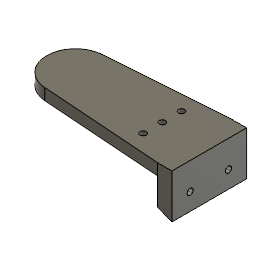
Femur 2 (Autodesk Fusion 360 design; units mm, degrees)
Autodesk Fusion 360 part; units mm, degrees
note: some values were not read from the file. Set by a fixed rule: which sketch regions a step uses.
sketch "Sketch1" plane through (0, 0, 0) normal (0, 1, 0) x (1, 0, 0)
  line L0 (-3.75, 19.5) -> (3.75, 19.5)
  line L1 (3.75, 19.5) -> (3.75, -19.5)
  line L2 (3.75, -19.5) -> (-3.75, -19.5)
  line L3 (-3.75, -19.5) -> (-3.75, 19.5)
  line L4 (-3.75, 19.5) -> (3.75, -19.5) construction
  line L5 (3.75, 19.5) -> (-3.75, -19.5) construction
  circle A0 centre (-66.05, 0) radius 15
  line L6 (-3.75, -19.5) -> (-67.1215, -14.9617)
  line L7 (-3.75, 19.5) -> (-67.1215, 14.9617)
  dimension "d1" = 7.5
  dimension "d2" = 39
  dimension "d4" = 30
  constraint horizontal L0
  constraint perpendicular L0 L1
  constraint parallel L0 L2
  constraint parallel L1 L3
  constraint coincident L4 origin
  constraint coincident L5 origin
  constraint tangent A0 L6
  constraint tangent A0 L7
  constraint coincident A0 L7.end
  constraint coincident A0 L6.end
  measures "d1" distance of L1.end L2.end
  measures "d2" distance of L0.end L1.end
  measures "d4" diameter of A0
extrude "Extrude1" add sketch "Sketch1" along normal blind 6
sketch "Sketch2" plane through (0, 6, 0) normal (0, 1, 0) x (-1, 0, 0)
  line L0 (-3.75, -19.5) -> (3.75, -19.5)
  line L1 (3.75, -19.5) -> (67.1215, -14.9617)
  arc A0 (67.1215, -14.9617) -> (67.1215, 14.9617) centre (66.05, 0) ccw
  line L2 (67.1215, 14.9617) -> (3.75, 19.5)
  line L3 (3.75, 19.5) -> (-3.75, 19.5)
  line L4 (-3.75, 19.5) -> (-3.75, -19.5)
  line L5 (-3.75, 19.5) -> (3.75, 19.5)
  line L6 (3.75, 19.5) -> (3.75, -19.5)
  line L7 (3.75, -19.5) -> (-3.75, -19.5)
  line L8 (-3.75, -19.5) -> (-3.75, 19.5)
  line L9 (-3.75, 19.5) -> (3.75, -19.5) construction
  line L10 (3.75, 19.5) -> (-3.75, -19.5) construction
  dimension "d7" = 7.5
  dimension "d8" = 39
  constraint horizontal L5
  constraint perpendicular L5 L6
  constraint parallel L5 L7
  constraint parallel L6 L8
  constraint coincident L9 origin
  constraint coincident L10 origin
  measures "d7" distance of L0.end L0.start
  measures "d8" distance of L2.end L0.end
extrude "Extrude2" add sketch "Sketch2" against normal blind 20.2 contours L0 L3 L4 L5 L6 L7 L8
sketch "Sketch3" plane through (0, 6, 0) normal (0, 1, 0) x (-1, 0, 0)
  line L0 (3.75, -19.5) -> (67.1215, -14.9617)
  arc A0 (67.1215, -14.9617) -> (67.1215, 14.9617) centre (66.05, 0) ccw
  line L1 (67.1215, 14.9617) -> (3.75, 19.5)
  line L2 (3.75, 19.5) -> (-3.75, 19.5)
  line L3 (-3.75, 19.5) -> (-3.75, -19.5)
  line L4 (-3.75, -19.5) -> (3.75, -19.5)
  circle A1 centre (66.05, 0) radius 4
  dimension "d11" = 8
  constraint concentric A0 A1
  measures "d11" diameter of A1
extrude "Extrude3" add sketch "Sketch3" against normal blind 9 contours A1
sketch "Sketch4" plane through (0, -3, 0) normal (0, -1, 0) x (1, 0, 0)
  circle A0 centre (-66.05, 0) radius 4
  circle A1 centre (-66.05, 0) radius 3
  dimension "d14" = 6
  constraint concentric A0 A1
  measures "d14" diameter of A1
extrude "Extrude4" add sketch "Sketch4" along normal blind 6 contours A1
sketch "Sketch5" plane through (0, 6, 0) normal (0, 1, 0) x (-1, 0, 0)
  line L0 (3.75, -19.5) -> (67.1215, -14.9617)
  arc A0 (67.1215, -14.9617) -> (67.1215, 14.9617) centre (66.05, 0) ccw
  line L1 (67.1215, 14.9617) -> (3.75, 19.5)
  line L2 (3.75, 19.5) -> (-3.75, 19.5)
  line L3 (-3.75, 19.5) -> (-3.75, -19.5)
  line L4 (-3.75, -19.5) -> (3.75, -19.5)
  line L5 (3.75, -19.5) -> (23.6989, -18.0714)
  line L6 (3.75, 19.5) -> (23.6989, 18.0714)
  line L7 (23.6989, 18.0714) -> (23.6989, -18.0714)
  line L8 (23.6989, -18.0714) -> (17.7142, -18.5)
  line L9 (23.6989, 18.0714) -> (17.7142, 18.5)
  line L10 (17.7142, 18.5) -> (17.7142, -18.5)
  line L11 (17.7142, -18.5) -> (23.6989, 18.0714)
  line L12 (23.6989, -18.0714) -> (17.7142, 18.5)
  line L13 (17.7142, 0) -> (23.6989, 0)
  circle A1 centre (20.7416, 0) radius 1.6
  line L14 (20.7416, 0) -> (20.7416, 10)
  circle A2 centre (20.7416, 10) radius 1.6
  line L15 (20.7416, 0) -> (20.7416, -10)
  circle A3 centre (20.7416, -10) radius 1.6
  dimension "d17" = 20
  dimension "d18" = 20
  dimension "d19" = 6
  dimension "d20" = 6
  dimension "d21" = 3.2
  dimension "d22" = 10
  dimension "d23" = 3.2
  dimension "d24" = 10
  dimension "d25" = 3.2
  constraint coincident L0.start L4.end
  constraint parallel L0 L5
  constraint coincident L1.end L2.start
  constraint parallel L1 L6
  constraint parallel L0 L8
  constraint parallel L1 L9
  constraint midpoint L10 L13.start
  constraint midpoint L7 L13.end
  constraint coincident L11 A1.centre
  constraint coincident L12 A1.centre
  constraint coincident A1.centre L14.start
  constraint perpendicular L13 L14
  constraint coincident L14.end A2.centre
  constraint perpendicular L13 L15
  constraint coincident L15.end A3.centre
  measures "d17" distance of L0.start L5.end
  measures "d18" distance of L1.end L6.end
  measures "d19" distance of L5.end L8.end
  measures "d20" distance of L6.end L9.end
  measures "d21" diameter of A1
  measures "d22" distance of A1.centre L14.end
  measures "d23" diameter of A2
  measures "d24" distance of A1.centre L15.end
  measures "d25" diameter of A3
extrude "Extrude5" cut sketch "Sketch5" against normal blind 13 contours L11 L13 A1 | L11 A1 L15 | L12 A1 L15 | L12 L13 A1 | L12 L13 A1 | L11 A1 L14 | L11 L13 A1 | L12 A1 L14 | A2 | A3
sketch "Sketch6" plane through (0, 0, 19.5) normal (0, 0, 1) x (1, 0, 0)
  line L0 (3.75, -14.2) -> (3.75, 6)
  line L1 (3.75, 6) -> (-3.75, 6)
  line L2 (-3.75, 6) -> (-3.75, 0)
  line L3 (-3.75, 0) -> (-3.75, -14.2)
  line L4 (-3.75, -14.2) -> (3.75, -14.2)
  line L5 (3.75, -14.2) -> (3.75, -17.07)
  line L6 (3.75, -17.07) -> (-3.75, -14.2)
  dimension "d28" = 2.87
  constraint coincident L0.start L4.end
  constraint perpendicular L4 L5
  constraint coincident L3.end L4.start
  measures "d28" distance of L0.start L5.end
extrude "Extrude6" add sketch "Sketch6" against normal blind 39 contours L4 L5 L6
sketch "Sketch7" plane through (-3.75, 0, 0) normal (-1, 0, 0) x (0, 0, 1)
  line L0 (19.5, 0) -> (-19.5, 0)
  line L1 (-19.5, 0) -> (-19.5, -14.2)
  line L2 (-19.5, -14.2) -> (19.5, -14.2)
  line L3 (19.5, -14.2) -> (19.5, 0)
  line L4 (-19.5, -14.2) -> (-10, -14.2)
  line L5 (-10, -14.2) -> (-10, -8.1)
  line L6 (-10, -8.1) -> (10, -8.1)
  circle A0 centre (-10, -8.1) radius 1.6
  circle A1 centre (10, -8.1) radius 1.6
  dimension "d31" = 9.5
  dimension "d32" = 6.1
  dimension "d33" = 20
  dimension "d34" = 3.2
  dimension "d35" = 3.2
  constraint coincident L1.end L2.start
  constraint perpendicular L1 L4
  constraint perpendicular L2 L5
  constraint perpendicular L5 L6
  constraint coincident L5.end L6.start
  constraint coincident L6.end A1.centre
  measures "d31" distance of L1.end L4.end
  measures "d32" distance of L4.end L5.end
  measures "d33" distance of L5.end L6.end
  measures "d34" diameter of A0
  measures "d35" diameter of A1
extrude "Extrude7" cut sketch "Sketch7" against normal blind 61 contours L5 L6 A0 | L5 L6 A0 | A1
